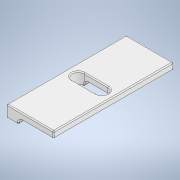
# Autodesk Inventor part: Carrier Clip V1
Saved by Autodesk Inventor 2022 (Build 260153000, 153)
## iProperties
Created: 2022-04-14
Part Number: Carrier Clip V1
Material: ABS Plastic
Document SubType Name: Modeling
Designer: Caleb
Density: 1.06 g/cm^3
Appearance: Smooth - White
Author: Caleb
Autodesk Inventor part; units mm, degrees
ref_plane "YZ Plane" through (0, 0, 0) normal (1, 0, 0) x (0, 1, 0)
ref_plane "XZ Plane" through (0, 0, 0) normal (0, 1, 0) x (-1, 0, 0)
ref_plane "XY Plane" through (0, 0, 0) normal (0, 0, 1) x (1, 0, 0)
sketch "Sketch1" plane through (0, 0, 0) normal (0, 1, 0) x (-1, 0, 0)
  line L0 (-9.525, -24.13) -> (9.525, -24.13)
  line L1 (9.525, -24.13) -> (9.525, 24.13)
  line L2 (9.525, 24.13) -> (-9.525, 24.13)
  line L3 (-9.525, 24.13) -> (-9.525, -24.13)
  line L4 (-9.525, -24.13) -> (9.525, 24.13) construction
  line L5 (9.525, -24.13) -> (-9.525, 24.13) construction
  point P0 (0, 0)
  dimension "d0" = 19.05
  dimension "d1" = 48.26
  constraints: 12 end point, 2 midpoint, 2 parallel, 1 horizontal, 1 perpendicular
  measures "d0" distance of L2.end L1.end
  measures "d1" distance of L0.end L1.end
extrude "Extrusion1" add sketch "Sketch1" along normal blind 4.7625
sketch "Sketch2" plane through (-9.525, 0, 24.13) normal (0, 0, 1) x (1, 0, 0)
  line L0 (19.05, 0) -> (19.05, 4.7625) projected
  line L1 (19.05, 2.1) -> (6.35, 2.1)
  line L2 (4.7625, 0.5125) -> (4.7625, 0)
  line L3 (0, 0) -> (19.05, 0) projected
  line L4 (0, 4.7625) -> (19.05, 4.7625) projected
  arc A0 (6.35, 2.1) -> (4.7625, 0.5125) centre (6.35, 0.5125) ccw
  point P0 (9.525, 0)
  point P1 (4.7625, 2.1)
  dimension "d4" = 14.2875
  dimension "d6" = 1.5875
  dimension "d21" = 2.1
  constraints: 4 end point, 4 point on line, 2 point on circle, 2 tangent, 1 centre point, 1 perpendicular, 1 vertical
  measures "d4" distance of L1.start point (4.763, 2.1)
  measures "d6" radius of A0
  measures "d21" distance between parallel lines of L3 L1
extrude "Extrusion2" cut sketch "Sketch2" against normal through all
sketch "Sketch3" plane through (-3.175, 2.1, 24.13) normal (0, -1, 0) x (1, 0, 0)
  line L0 (1.4801, -24.13) -> (10.1501, -24.13)
  line L1 (12.7, 0) -> (12.7, -48.26) projected
  circle A0 centre (9.525, -4.33) radius 1.1
  circle A1 centre (9.525, -43.93) radius 1.1
  point P0 (3.175, -24.13)
  dimension "d9" = 39.6
  dimension "d10" = 3.175
  dimension "d11" = 2.2
  dimension "d12" = 2.2
  constraints: 2 centre point, 2 coincident, 2 end point, 1 horizontal, 1 point on line, 1 symmetric about line, 1 vertical alignment
  measures "d9" distance of point (9.525, -4.33) point (9.525, -43.93)
  measures "d10" distance from line of L1 point (9.525, -4.33)
  measures "d11" diameter of A0
  measures "d12" diameter of A1
extrude "Extrusion3" add sketch "Sketch3" along normal blind 1.5875
fillet "Fillet1" radius 0.7937 2 edges at (5.25, 0.5125, 19.8) (5.25, 0.5125, -19.8)
sketch "Sketch4" plane through (0, 4.7625, 0) normal (0, 1, 0) x (1, 0, 0)
  line L0 (4.7625, 0) -> (-4.7625, 0) construction
  line L1 (-3.175, -24.13) -> (-3.175, 24.13) projected
  line L2 (4.7625, 2.3813) -> (-4.7625, 2.3812)
  line L3 (-4.7625, -2.3813) -> (4.7625, -2.3813)
  arc A0 (4.7625, -2.3813) -> (4.7625, 2.3813) centre (4.7625, 0) ccw
  arc A1 (-4.7625, 2.3812) -> (-4.7625, -2.3813) centre (-4.7625, 0) ccw
  line L4 (-9.525, 24.13) -> (-9.525, -24.13) projected
  point P0 (0, 0)
  point P1 (0, 0)
  dimension "d16" = 2.3813
  dimension "d17" = 9.525
  dimension "d18" = 9.525
  constraints: 8 end point, 4 point on circle, 4 tangent, 2 centre point, 1 midpoint, 1 parallel, 1 perpendicular
  measures "d16" radius of A1
  measures "d17" distance of L3.start L3.end
  measures "d18" distance from line of L4 point (0, 0)
extrude "Extrusion4" cut sketch "Sketch4" against normal through all
fillet "Fillet2" radius 0.3969 30 edges at (3.175, 2.1, 24.13) (-4.7625, 0.2562, 24.13) (-4.2975, 1.635, 24.13) (-7.1437, 0, 24.13) (-4.7625, 0, 13.2556) (-4.7625, 0, -13.2556) (9.525, 2.1, 0) (-9.525, 0, 0) (-9.525, 2.3813, 24.13) (-9.525, 2.3813, -24.13) (-7.1437, 0, -24.13) (-4.2975, 1.635, -24.13) (-4.7625, 0.2562, -24.13) (3.175, 2.1, -24.13) (-7.1438, 0, 0) (0.7938, 2.1, 2.3813) (7.1438, 2.1, 0) (0.7938, 2.1, -2.3812) (-4.2975, 1.635, -2.3812) (-4.2975, 1.635, 2.3813) (9.525, 3.4313, -24.13) (9.525, 3.4313, 24.13) (9.525, 4.7625, 0) (0, 4.7625, 24.13) (0, 4.7625, 2.3813) (-7.1438, 4.7625, 0) (0, 4.7625, -2.3812) (7.1438, 4.7625, 0) (0, 4.7625, -24.13) (-9.525, 4.7625, 0)
equation "\"d12\" = d11"
body "Solid1"
